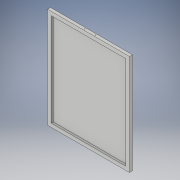
# Autodesk Inventor part: WoodFrame
Saved by Autodesk Inventor 2019 (Build 230136000, 136)
## iProperties
Created: 2018-10-04
Part Number: WoodFrame
Material: Generic
Document SubType Name: Modeling
Designer: abhay
Density: 1 g/cm^3
Appearance: Default
Author: abhay
Autodesk Inventor part; units mm, degrees
ref_plane "YZ Plane" through (0, 0, 0) normal (1, 0, 0) x (0, 1, 0)
ref_plane "XZ Plane" through (0, 0, 0) normal (0, 1, 0) x (-1, 0, 0)
ref_plane "XY Plane" through (0, 0, 0) normal (0, 0, 1) x (1, 0, 0)
sketch "Sketch1" plane through (0, 0, 0) normal (0, 0, 1) x (1, 0, 0)
  line L0 (-275, -337.5) -> (275, -337.5)
  line L1 (275, -337.5) -> (275, 337.5)
  line L2 (275, 337.5) -> (-275, 337.5)
  line L3 (-275, 337.5) -> (-275, -337.5)
  line L4 (-275, -337.5) -> (275, 337.5) construction
  line L5 (275, -337.5) -> (-275, 337.5) construction
  point P0 (0, 0)
  dimension "d0" = 550
  dimension "d1" = 675
  constraints: 12 end point, 2 midpoint, 2 parallel, 1 horizontal, 1 perpendicular
  measures "d0" distance of L2.end L1.end
  measures "d1" distance of L1.end L0.end
extrude "Extrusion1" add sketch "Sketch1" along normal blind 20
sketch "Sketch2" plane through (0, 0, 20) normal (0, 0, 1) x (1, 0, 0)
  line L0 (-250, -312.5) -> (250, -312.5)
  line L1 (250, -312.5) -> (250, 312.5)
  line L2 (250, 312.5) -> (-250, 312.5)
  line L3 (-250, 312.5) -> (-250, -312.5)
  line L4 (-250, -312.5) -> (250, 312.5) construction
  line L5 (250, -312.5) -> (-250, 312.5) construction
  point P0 (0, 0)
  dimension "d4" = 500
  dimension "d5" = 625
  constraints: 12 end point, 2 midpoint, 2 parallel, 1 horizontal, 1 perpendicular
  measures "d4" distance of L2.end L1.end
  measures "d5" distance of L1.end L0.end
extrude "Extrusion2" cut sketch "Sketch2" against normal blind 13
sketch "Sketch3" plane through (-275, 337.5, 0) normal (0, 1, 0) x (1, 0, 0)
  line L0 (550, 0) -> (550, -20) projected
  line L1 (0, 0) -> (0, -20) projected
  line L2 (0, 0) -> (0, -20) projected
  line L3 (0, -10) -> (230.6764, -10)
  line L4 (525, -7) -> (25, -7) projected
  line L5 (0, -10) -> (230.6764, -10) construction
  line L6 (319.3236, 0) -> (230.6764, 0)
  line L7 (230.6764, 0) -> (230.6764, -20)
  line L8 (230.6764, -20) -> (319.3236, -20)
  line L9 (319.3236, -20) -> (319.3236, 0)
  line L10 (319.3236, 0) -> (230.6764, -20) construction
  line L11 (230.6764, 0) -> (319.3236, -20) construction
  circle A0 centre (239.2871, -10) radius 2.1828
  line L12 (275, 0) -> (275, -20)
  circle A1 centre (310.7129, -10) radius 2.1828
  point P0 (275, -10)
  dimension "d8" = 550
  dimension "d9" = 230.6764
  dimension "d10" = 0
  dimension "d11" = 4.3656
  dimension "d12" = 8.6106
  constraints: 18 end point, 4 midpoint, 4 parallel, 2 centre point, 1 collinear, 1 horizontal, 1 perpendicular, 1 symmetric about line, 1 other
  measures "d8" distance between parallel lines of L0 L1
  measures "d9" distance of L3.start L3.end
  measures "d10" distance between parallel lines of L3 L5
  measures "d11" diameter of A0
  measures "d12" distance from line of L7 A0.centre
extrude "Extrusion3" cut sketch "Sketch3" against normal blind 15 contours A0 | A1
body "Solid1"
